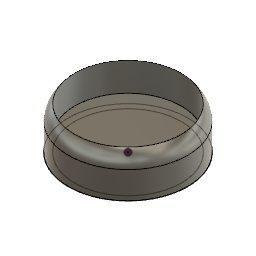
Clothes Stand Foot (Autodesk Fusion 360 design; units mm, degrees)
Autodesk Fusion 360 part; units mm, degrees
sketch "Sketch1" plane through (0, 0, 0) normal (0, 1, 0) x (1, 0, 0)
  circle A0 centre (0, 0) radius 12.65
  circle A1 centre (0, 0) radius 14.15
  dimension "d1" = 25.3
  dimension "d2" = 28.3
  constraint coincident A0.centre A1.centre
  constraint concentric A0 A1
  measures "d1" diameter of A0
  measures "d2" diameter of A1
extrude "Extrude1" add sketch "Sketch1" along normal blind 10 contours A0 | A1
extrude "Extrude2" cut sketch "Sketch1" along normal blind 10 from surface at 3.2 contours A0
fillet "Fillet1" radius 5 1 edges at (-13.1924, 10, 5.1169)
